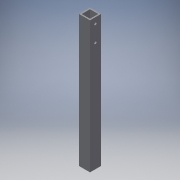
# Autodesk Inventor part: Substitute Sucker Arm
Saved by Autodesk Inventor 2017 (Build 210142000, 142)
## iProperties
Created: 2016-10-01
Part Number: Substitute Sucker Arm
Material: Generic
Document SubType Name: Modeling
Designer: 15102898
Density: 1 g/cm^3
Appearance: Default
Author: 15102898
Autodesk Inventor part; units mm, degrees
ref_plane "YZ Plane" through (0, 0, 0) normal (1, 0, 0) x (0, 1, 0)
ref_plane "XZ Plane" through (0, 0, 0) normal (0, 1, 0) x (-1, 0, 0)
ref_plane "XY Plane" through (0, 0, 0) normal (0, 0, 1) x (1, 0, 0)
sketch "Sketch1" plane through (0, 0, 0) normal (0, 1, 0) x (-1, 0, 0)
  line L0 (0, 0) -> (25.4, 0)
  line L1 (25.4, 0) -> (25.4, 25.4)
  line L2 (25.4, 25.4) -> (0, 25.4)
  line L3 (0, 25.4) -> (0, 0)
  line L4 (3.175, 22.225) -> (22.225, 22.225)
  line L5 (22.225, 22.225) -> (22.225, 3.175)
  line L6 (22.225, 3.175) -> (3.175, 3.175)
  line L7 (3.175, 3.175) -> (3.175, 22.225)
  dimension "d0" = 25.4
  dimension "d1" = 25.4
  dimension "d4" = 3.175
  dimension "d5" = 3.175
  dimension "d6" = 3.175
  dimension "d7" = 3.175
  constraints: 16 end point, 4 parallel, 2 horizontal, 2 perpendicular
  measures "d0" distance of L2.end L1.end
  measures "d1" distance of L1.end L0.end
  measures "d4" distance between parallel lines of L1 L5
  measures "d5" distance between parallel lines of L0 L6
  measures "d6" distance between parallel lines of L3 L7
  measures "d7" distance between parallel lines of L2 L4
extrude "Extrusion1" add sketch "Sketch1" along normal blind 304.8
sketch "Sketch2" plane through (0, 0, 25.4) normal (1, 0, 0) x (0, 0, -1)
  circle A0 centre (12.7, 292.1) radius 3.175
  line L0 (22.225, 304.8) -> (3.175, 304.8) projected
  line L1 (0, 0) -> (0, 304.8) projected
  point P0 (25.4, 0)
  dimension "d10" = 6.35
  dimension "d11" = 12.7
  dimension "d12" = 12.7
  constraints: 1 centre point
  measures "d10" diameter of A0
  measures "d11" distance from line of L0 A0.centre
  measures "d12" distance from line of L1 A0.centre
extrude "Extrusion2" cut sketch "Sketch2" against normal blind 304.8
sketch "Sketch3" plane through (-25.4, 0, 0) normal (-1, 0, 0) x (0, 0, 1)
  circle A0 centre (12.7, 254) radius 3.175
  line L0 (0, 304.8) -> (25.4, 304.8) projected
  line L1 (0, 0) -> (0, 304.8) projected
  dimension "d15" = 6.35
  dimension "d16" = 50.8
  dimension "d17" = 12.7
  constraints: 1 centre point
  measures "d15" diameter of A0
  measures "d16" distance from line of L0 A0.centre
  measures "d17" distance from line of L1 A0.centre
extrude "Extrusion3" cut sketch "Sketch3" against normal blind 25.4
sketch "Sketch4" plane through (-25.4, 0, 25.4) normal (0, 0, 1) x (1, 0, 0)
  line L0 (11.9432, 247.65) -> (11.9432, 304.8) construction
  line L1 (21.4682, 247.65) -> (21.4682, 304.8)
  line L2 (2.4182, 304.8) -> (2.4182, 247.65)
  arc A0 (2.4182, 247.65) -> (21.4682, 247.65) centre (11.9432, 247.65) ccw
  arc A1 (21.4682, 304.8) -> (2.4182, 304.8) centre (11.9432, 304.8) ccw
  line L3 (0, 0) -> (25.4, 0) projected
  line L4 (0, 0) -> (0, 304.8) projected
  line L5 (22.225, 304.8) -> (3.175, 304.8) projected
  point P0 (11.9432, 276.225)
  dimension "d20" = 57.15
  dimension "d22" = 11.9432
  dimension "d23" = 0
  dimension "d24" = 19.05
  constraints: 8 end point, 4 point on circle, 4 tangent, 2 centre point, 1 midpoint, 1 parallel, 1 vertical
  measures "d20" distance of L0.start L0.end
  measures "d22" distance from line of L4 L0.end
  measures "d23" distance from line of L5 L0.end
  measures "d24" distance between parallel lines of L1 L2
extrude "Extrusion4" cut sketch "Sketch4" against normal blind 3.175
equation "\"d5\" = d4"
equation "\"d6\" = d4"
equation "\"d7\" = d4"
body "Solid1"
